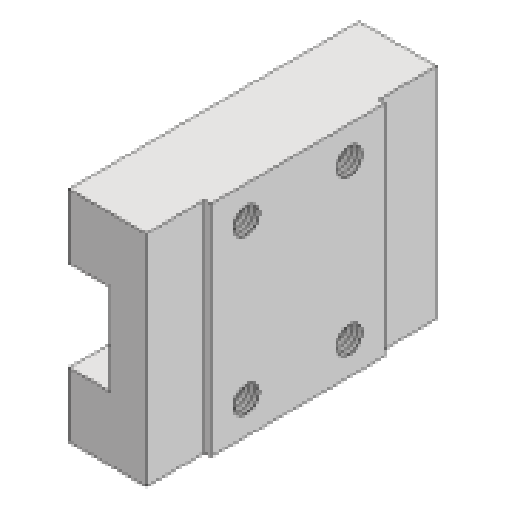
# Autodesk Inventor part: mgn7c carrige
Saved by Autodesk Inventor 2023 (Build 270158000, 158)
## iProperties
Created: 2022-10-31
Part Number: mgn7c carrige
Material: Generic
Document SubType Name: Modeling
Designer: deli
Density: 1 g/cm^3
Appearance: Default
Author: deli
Autodesk Inventor part; units mm, degrees
ref_plane "YZ Plane" through (0, 0, 0) normal (1, 0, 0) x (0, 1, 0)
ref_plane "XZ Plane" through (0, 0, 0) normal (0, 1, 0) x (-1, 0, 0)
ref_plane "XY Plane" through (0, 0, 0) normal (0, 0, 1) x (1, 0, 0)
sketch "Sketch1" plane through (0, 0, 0) normal (0, 0, 1) x (1, 0, 0)
  line L0 (69.9988, 111.2194) -> (69.9988, 106.2194)
  line L1 (69.9988, 106.2194) -> (73.1128, 106.2194)
  line L2 (73.1128, 106.2194) -> (73.1128, 99.2194)
  line L3 (73.1128, 99.2194) -> (69.9988, 99.2194)
  line L4 (69.9988, 99.2194) -> (69.9988, 94.2194)
  line L5 (69.9988, 94.2194) -> (76.4988, 94.2194)
  line L6 (76.4988, 94.2194) -> (76.4988, 111.2194)
  line L7 (76.4988, 111.2194) -> (69.9988, 111.2194)
  point P0 (0, 0)
  dimension "d1" = 17
  dimension "d2" = 7
  dimension "d3" = 6.5
  constraints: 16 end point, 6 perpendicular, 2 point on line, 1 collinear, 1 vertical
  measures "d1" distance of L5.end L6.end
  measures "d2" distance of L1.end L2.end
  measures "d3" distance of L6.end L0.start
extrude "Extrusion1" add sketch "Sketch1" along normal blind 22.5
sketch "Sketch2" plane through (76.4988, 94.2194, 0) normal (1, 0, 0) x (0, 0, -1)
  line L0 (-22.5, 0) -> (-22.5, 17) projected
  line L1 (-22.5, 17) -> (-18, 17)
  line L2 (-18, 17) -> (-18, 0)
  line L3 (-18, 0) -> (-22.5, 0)
  line L4 (-22.5, 0) -> (-22.5, 17)
  line L5 (0, 17) -> (-22.5, 17) projected
  line L6 (0, 17) -> (-4.5, 17)
  line L7 (-4.5, 17) -> (-4.5, 0)
  line L8 (-4.5, 0) -> (0, 0)
  line L9 (0, 0) -> (0, 17)
  point P0 (0, -94.2194)
  dimension "d6" = 13.5
  dimension "d7" = 4.5
  dimension "d8" = 22.5
  constraints: 16 end point, 4 parallel, 2 horizontal, 2 perpendicular
  measures "d6" distance between parallel lines of L7 L2
  measures "d7" distance between parallel lines of L2 L0
  measures "d8" distance between parallel lines of L9 L0
extrude "Extrusion2" cut sketch "Sketch2" against normal blind 0.5
sketch "Sketch3" plane through (76.4988, 94.2194, 4.5) normal (1, 0, 0) x (0, 0, -1)
  circle A0 centre (-10.75, 14.5) radius 1
  circle A1 centre (-2.75, 14.5) radius 1
  circle A2 centre (-10.75, 2.5) radius 1
  circle A3 centre (-2.75, 2.5) radius 1
  line L0 (-10.75, 14.5) -> (-2.75, 14.5) construction
  line L1 (-2.75, 14.5) -> (-2.75, 2.5) construction
  line L2 (-2.75, 2.5) -> (-10.75, 2.5) construction
  line L3 (-10.75, 2.5) -> (-10.75, 14.5) construction
  line L4 (0, 17) -> (-13.5, 17) construction
  line L5 (-13.5, 17) -> (-13.5, 0) construction
  point P0 (4.5, -94.2194)
  dimension "d11" = 2
  dimension "d12" = 8
  dimension "d13" = 12
  dimension "d14" = 2.5
  dimension "d15" = 2.75
  dimension "d16" = 13.5
  dimension "d17" = 17
  constraints: 8 end point, 4 centre point, 3 equal radius, 3 perpendicular, 1 horizontal
  measures "d11" diameter of A0
  measures "d12" distance of L0.start L0.end
  measures "d13" distance of L2.end L0.start
  measures "d14" distance between parallel lines of L4 L0
  measures "d15" distance between parallel lines of L5 L3
  measures "d16" distance of L4.start L4.end
  measures "d17" distance of L4.end L5.end
extrude "Extrusion3" cut sketch "Sketch3" against normal blind 6
thread "Thread1" size "M2x0.4" class "6H" standard "ANSI Metric M Profile" full length
thread "Thread2" size "M2x0.4" class "6H" standard "ANSI Metric M Profile" full length
thread "Thread3" size "M2x0.4" class "6H" standard "ANSI Metric M Profile" full length
thread "Thread4" size "M2x0.4" class "6H" standard "ANSI Metric M Profile" full length
equation "\"d7\" = -0.5 * d6 + 0.5 * d8"
equation "\"d14\" = -0.5 * d13 + 0.5 * d17"
equation "\"d15\" = -0.5 * d12 + 0.5 * d16"
body "Solid1"
